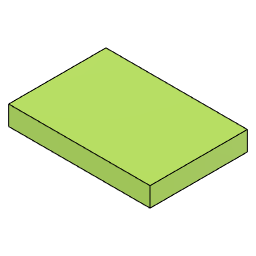
Chest v10 (Autodesk Fusion 360 archive; units mm, degrees)
design "Chest" references "Head V2 - OBS"
Autodesk Fusion 360 part; units mm, degrees
sketch "Sketch1" plane through (0, 0, 0) normal (0, 1, 0) x (1, 0, 0)
  line L0 (109, 75) -> (-109, 75)
  line L1 (-109, 75) -> (-109, -75)
  line L2 (-109, -75) -> (109, -75)
  line L3 (109, -75) -> (109, 75)
  line L4 (109, 75) -> (-109, -75) construction
  line L5 (-109, 75) -> (109, -75) construction
  dimension "d1" = 218
  dimension "d2" = 150
  constraint horizontal L0
  constraint perpendicular L0 L1
  constraint parallel L0 L2
  constraint parallel L1 L3
  constraint coincident L4 origin
  constraint coincident L5 origin
  measures "d1" distance of L1.end L2.end
  measures "d2" distance of L0.end L1.end
extrude "Extrude1" add sketch "Sketch1" along normal mid plane 30
move_body "Move1" [suppressed]
moveface "MoveFace1" [suppressed]
move_body "Move2" [suppressed]
move_body "Move3" [suppressed]
move_body "Move4" [suppressed]
move_body "Move5" [suppressed]
move_body "Move6" [suppressed]
move_body "Move7" [suppressed]
moveface "MoveFace2" [suppressed]
moveface "MoveFace3" [suppressed]
move_body "Move8" [suppressed]
moveface "MoveFace4" [suppressed]
move_body "Move9" [suppressed]
sketch "Sketch2" plane through (0, 0, 0) normal (1, 0, 0) x (0, 0, -1)
  circle A0 centre (-396.6427, 621.3445) radius 33.0645
  point P0 (-474.3324, 127.4171)
move_body "Move11" [suppressed]
